Autodesk Inventor part; units mm, degrees
note: some values were not read from the file. Chosen so that the rebuilt part matches the saved one: direction of "Hole2".
(part 18 of 18)
sketch "Sketch18" plane through (0, 13.762, -10) normal (0, 1, 0) x (1, 0, 0)
  line L0 (-9.984, -13.984) -> (-9.984, 28.9609) projected
  line L1 (-9.984, 28.9609) -> (9.984, 28.9609) projected
  line L2 (9.984, 28.9609) -> (9.984, -13.984) projected
  line L3 (9.984, -13.984) -> (-9.984, -13.984) projected
  line L4 (11, -15) -> (11, 29.9769) projected
  line L5 (11, 29.9769) -> (-11, 29.9769) projected
  line L6 (-11, 29.9769) -> (-11, -15) projected
  line L7 (-11, -15) -> (11, -15) projected
  point P0 (0, -10)
extrude "Extrusion13" add sketch "Sketch18" along normal blind 11.5 draft 6
sketch "Sketch19" plane through (0, 25.262, -10) normal (0, 1, 0) x (1, 0, 0)
  line L0 (-10.6847, 29.1856) -> (10.5796, 29.1856)
  line L1 (10.5796, 29.1856) -> (10.5796, -14.6847)
  line L2 (10.5796, -14.6847) -> (-10.6847, -14.6847)
  line L3 (-10.6847, -14.6847) -> (-10.6847, 29.1856)
  line L4 (-12.2087, 31.1856) -> (12.2087, 31.1856) projected
  line L5 (12.2087, -16.2087) -> (-12.2087, -16.2087) projected
  line L6 (-12.2087, -16.2087) -> (-12.2087, 31.1856) projected
  point P0 (0, -10)
  point P1 (-0.0526, 29.1856)
  point P2 (-0.0526, 28.3136)
  dimension "d183" = 2
  dimension "d184" = 1.524
  dimension "d185" = 1.524
  constraints: 8 end point, 2 parallel, 1 horizontal, 1 midpoint, 1 perpendicular, 1 vertical alignment
  measures "d183" distance between parallel lines of L0 L4
  measures "d184" distance between parallel lines of L5 L2
  measures "d185" distance between parallel lines of L3 L6
sketch "Sketch20" plane through (0, 13.762, -10) normal (0, 1, 0) x (-1, 0, 0)
  line L0 (9.984, 13.984) -> (-9.984, 13.984)
  line L1 (-9.984, 13.984) -> (-9.984, -28.9609)
  line L2 (-9.984, -28.9609) -> (9.984, -28.9609)
  line L3 (9.984, -28.9609) -> (9.984, 13.984)
  point P0 (0, 10)
  constraints: 8 end point, 2 parallel, 1 coincident, 1 horizontal, 1 perpendicular
loft "Loft1" cut profiles "Sketch20", "Sketch19"
sketch "Sketch21" plane through (0, 25.262, -10) normal (0, 1, 0) x (1, 0, 0)
  line L0 (12.2087, 31.1856) -> (12.2087, -16.2087) projected
  line L1 (11, 29.9769) -> (-11, 29.9769) projected
  line L2 (-12.2087, 31.1856) -> (12.2087, 31.1856)
  line L3 (12.2087, 31.1856) -> (12.2087, 30.3448)
  line L4 (12.2087, 30.3448) -> (-12.2087, 30.3448)
  line L5 (-12.2087, 30.3448) -> (-12.2087, 31.1856)
  point P0 (0, -10)
  constraints: 8 end point, 2 parallel, 1 horizontal, 1 perpendicular, 1 point on line
extrude "Extrusion14" [suppressed]
ref_plane "Work Plane11" through (0, 0, -53) normal (0, 0, -1) x (-1, 0, 0)
sketch "Sketch29" plane through (2.9474, 25.262, -39.1856) normal (0, 0.9876883, 0.1564345) x (1, 0, 0)
  line L0 (-19.8442, 3.8517) -> (23.6634, 3.8517)
  line L1 (23.6634, 3.8517) -> (23.6634, -48.2313)
  line L2 (23.6634, -48.2313) -> (-19.8442, -48.2313)
  line L3 (-19.8442, -48.2313) -> (-19.8442, 3.8517)
  point P0 (0, 0)
  constraints: 8 end point, 2 parallel, 1 horizontal, 1 perpendicular
extrude "Extrusion16" cut sketch "Sketch29" along normal through all
sketch "Sketch31" plane through (2.9474, 25.262, -39.1856) normal (0, 0.9876883, 0.1564345) x (1, 0, 0)
  line L0 (8.518, -45.2076) -> (-14.4128, -45.2076) projected
  line L1 (-14.4128, -45.2076) -> (-15.1561, 0) projected
  line L2 (-13.6633, 0.9594) -> (7.6633, 0.9594)
  line L3 (7.6633, 0.9594) -> (7.6633, -44.4456)
  line L4 (7.6633, -44.4456) -> (-13.6633, -44.4456)
  line L5 (-13.6633, -44.4456) -> (-13.6633, 0.9594)
  line L6 (-2.9474, 132.6833) -> (-2.9474, -156.7902) projected
  line L7 (-13.6321, 0) -> (7.6321, 0) projected
  line L8 (-15.1561, 1.9754) -> (9.2613, 1.9754) projected
  point P0 (-2.9474, -42.655)
  point P1 (-3, 0.9594)
  point P2 (-3, 0)
  dimension "d198" = 1.016
  dimension "d199" = 0.762
  dimension "d200" = 0.762
  constraints: 8 end point, 2 midpoint, 2 parallel, 1 horizontal, 1 perpendicular, 1 vertical alignment
  measures "d198" distance between parallel lines of L2 L8
  measures "d199" distance between parallel lines of L0 L4
  measures "d200" distance from line of L4.end L1
extrude "Extrusion18" cut sketch "Sketch31" against normal blind 0.508
equation "\"d22\" = d24"
equation "\"d23\" = d24"
equation "\"d37\" = t"
equation "\"d40\" = t"
equation "\"t\" = 1.016"
equation "\"d14\" = d24"
equation "\"d24\" = 1.016"
body "Solid1"
